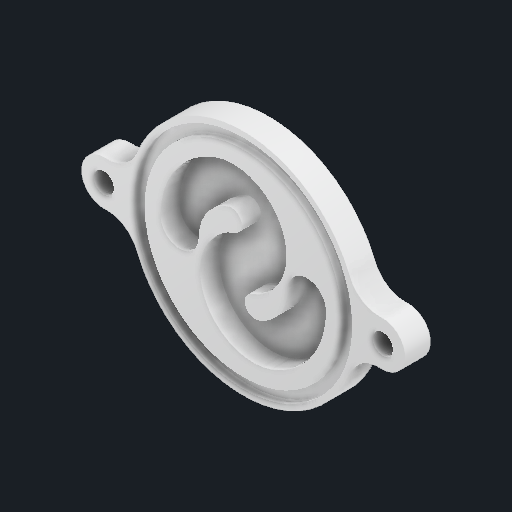
# Autodesk Inventor part: nema 14 heatsink
Saved by Autodesk Inventor 2024.3 (Build 283343000, 343)
## iProperties
Created: 2024-10-05
Part Number: nema 14 heatsink
Material: Aluminum 6061
Document SubType Name: Modeling
Designer: MFil
Density: 2.7 g/cm^3
Appearance: Aluminum - Flat
Mass: 8.37074 g
Surface Area: 34.2481 cm^2
Volume: 3.10027 cm^3
Author: MFil
Autodesk Inventor part; units mm, degrees
ref_plane "YZ Plane" through (0, 0, 0) normal (1, 0, 0) x (0, 1, 0)
ref_plane "XZ Plane" through (0, 0, 0) normal (0, 1, 0) x (-1, 0, 0)
ref_plane "XY Plane" through (0, 0, 0) normal (0, 0, 1) x (1, 0, 0)
sketch "Sketch1" plane through (0, 0, 0) normal (0, 0, 1) x (1, 0, 0)
  circle A0 centre (21.92, -18.1) radius 2.75 projected
  circle A1 centre (-21.92, -18.1) radius 1.8 projected
  circle A2 centre (21.92, -18.1) radius 3.5
  circle A3 centre (-21.92, -18.1) radius 3.5
  circle A4 centre (0, -18.1) radius 1.48 projected
  circle A5 centre (0, -18.1) radius 18
  circle A6 centre (21.3786, -26.5827) radius 5
  circle A7 centre (21.3786, -9.6173) radius 5
  circle A8 centre (-21.3786, -9.6173) radius 5
  circle A9 centre (-21.3786, -26.5827) radius 5
  circle A10 centre (21.92, -18.1) radius 1.6
  circle A11 centre (-21.92, -18.1) radius 1.6
  point P0 (0, 0)
  point P1 (21.6971, -14.6071)
  point P2 (16.7311, -11.4613)
  point P3 (-16.7311, -11.4613)
  point P4 (-21.6971, -14.6071)
  point P5 (-21.6971, -21.5929)
  point P6 (-16.7311, -24.7387)
  point P7 (16.7311, -24.7387)
  point P8 (21.6971, -21.5929)
  dimension "d0" = 7
  dimension "d1" = 7
  dimension "d2" = 36
  dimension "d3" = 10
  dimension "d4" = 10
  dimension "d5" = 10
  dimension "d6" = 10
  dimension "d7" = 3.2
  dimension "d8" = 3.2
  constraints: 9 centre point, 8 tangent, 5 coincident
  measures "d0" diameter of A2
  measures "d1" diameter of A3
  measures "d2" diameter of A5
  measures "d3" diameter of A6
  measures "d4" diameter of A7
  measures "d5" diameter of A8
  measures "d6" diameter of A9
  measures "d7" diameter of A10
  measures "d8" diameter of A11
extrude "Extrusion1" add sketch "Sketch1" along normal blind 1 contours A0 | A1 | A2 | A2 A6 A5 A7 | A5 | A5 A9 A3 A8 | A3 | A4
sketch "Sketch2" plane through (0, 0, 1) normal (0, 0, 1) x (1, 0, 0)
  arc A0 (16.7311, -11.4613) -> (21.6971, -14.6071) centre (21.3786, -9.6173) ccw projected
  arc A1 (16.7311, -11.4613) -> (-16.7311, -11.4613) centre (0, -18.1) ccw projected
  arc A2 (-21.6971, -14.6071) -> (-16.7311, -11.4613) centre (-21.3786, -9.6173) ccw projected
  arc A3 (-21.6971, -14.6071) -> (-21.6971, -21.5929) centre (-21.92, -18.1) ccw projected
  arc A4 (-16.7311, -24.7387) -> (-21.6971, -21.5929) centre (-21.3786, -26.5827) ccw projected
  arc A5 (-16.7311, -24.7387) -> (16.7311, -24.7387) centre (0, -18.1) ccw projected
  arc A6 (21.6971, -21.5929) -> (16.7311, -24.7387) centre (21.3786, -26.5827) ccw projected
  arc A7 (21.6971, -21.5929) -> (21.6971, -14.6071) centre (21.92, -18.1) ccw projected
  circle A8 centre (-21.92, -18.1) radius 1.6 projected
  circle A9 centre (21.92, -18.1) radius 1.6 projected
  circle A10 centre (0, -18.1) radius 18
  circle A11 centre (0, -18.1) radius 17.1
  circle A12 centre (0, -18.1) radius 15.5
  circle A13 centre (0, -18.1) radius 14.5
  point P0 (0, 0)
  dimension "d11" = 0.9
  dimension "d12" = 1.6
  dimension "d13" = 1
  constraints: 4 centre point, 1 coincident, 1 concentric
  measures "d11" radial gap between concentric circles of A10 A11
  measures "d12" radial gap between concentric circles of A11 A12
  measures "d13" radial gap between concentric circles of A12 A13
extrude "Extrusion2" add sketch "Sketch2" along normal blind 2 contours A10 A5 A1 | A0 A7 A6 A10 | A10 A4 A3 A2 | A11 | A12
extrude "Extrusion3" add sketch "Sketch2" along normal blind 3
sketch "Sketch3" plane through (0, -18.1, 1) normal (0, 0, 1) x (1, 0, 0)
  circle A0 centre (-10, 0) radius 3
  circle A1 centre (10, 0) radius 3
  circle A2 centre (0, 0) radius 14.5 projected
  arc A3 (-4.4463, 12.216) -> (-13, 0) centre (0, 0) ccw
  line L0 (0, 0) -> (-4.4463, 12.216) construction
  line L1 (0, 0) -> (-13, 0) construction
  arc A4 (4.4463, -12.216) -> (13, 0) centre (0, 0) ccw
  line L2 (0, 0) -> (4.4463, -12.216) construction
  line L3 (0, 0) -> (13, 0) construction
  arc A5 (-2.3941, 6.5778) -> (-7, 0) centre (0, 0) ccw
  line L4 (0, 0) -> (-2.3941, 6.5778) construction
  line L5 (0, 0) -> (-7, 0) construction
  arc A6 (2.3941, -6.5778) -> (7, 0) centre (0, 0) ccw
  line L6 (0, 0) -> (2.3941, -6.5778) construction
  line L7 (0, 0) -> (7, 0) construction
  arc A7 (1.2807, -3.5186) -> (-4.4463, 12.216) centre (-1.5828, 4.3487) ccw
  arc A8 (-1.2807, 3.5186) -> (-2.3941, 6.5778) centre (-1.8374, 5.0482) ccw
  arc A9 (1.2807, -3.5186) -> (2.3941, -6.5778) centre (1.8374, -5.0482) ccw
  arc A10 (-1.2807, 3.5186) -> (4.4463, -12.216) centre (1.5828, -4.3487) ccw
  point P0 (1.1789, -2.7195)
  dimension "d36" = 70
  dimension "d37" = 70
  dimension "d38" = 70
  dimension "d39" = 70
  dimension "d49" = 1
  constraints: 20 point on circle, 16 end point, 10 centre point, 5 coincident, 4 tangent, 2 equal radius, 1 horizontal alignment, 1 point on line, 6 other
  measures "d36" angle of L0 L1
  measures "d37" angle of L2 L3
  measures "d38" angle of L4 L5
  measures "d39" angle of L6 L7
extrude "Extrusion4" add sketch "Sketch3" along normal up to surface (3 mm away)
equation "\"d36\" = d37"
equation "\"d38\" = d39"
body "Solid1"
